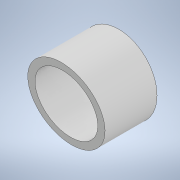
# Autodesk Inventor part: 20220612_仮筒
Saved by Autodesk Inventor 2020 (Build 240168000, 168)
## iProperties
Created: 2022-06-12
Part Number: 20220612_仮筒
Material: 一般
Document SubType Name: Modeling
Designer: Naggy
Density: 1 g/cm^3
Appearance: 既定
Author: Naggy
Autodesk Inventor part; units mm, degrees
ref_plane "YZ Plane" through (0, 0, 0) normal (1, 0, 0) x (0, 1, 0)
ref_plane "XZ Plane" through (0, 0, 0) normal (0, 1, 0) x (-1, 0, 0)
ref_plane "XY Plane" through (0, 0, 0) normal (0, 0, 1) x (1, 0, 0)
sketch "スケッチ1" plane through (0, 0, 0) normal (0, 0, 1) x (1, 0, 0)
  circle A0 centre (0, 0) radius 40
  dimension "d0" = 80
  constraints: 1 centre point, 1 coincident
  measures "d0" diameter of A0
extrude "押し出し1" add sketch "スケッチ1" along normal blind 60
sketch "スケッチ2" plane through (0, 0, 60) normal (0, 0, 1) x (1, 0, 0)
  circle A0 centre (0, 0) radius 32.5
  dimension "d3" = 65
  constraints: 1 centre point, 1 coincident
  measures "d3" diameter of A0
extrude "押し出し2" cut sketch "スケッチ2" against normal blind 60
sketch "スケッチ3" plane through (0, 0, 0) normal (1, 0, 0) x (0, 1, 0)
  line L0 (40, 0) -> (40, 60) projected
  line L1 (40, 60) -> (-40, 49.2831)
  line L2 (-40, 0) -> (-40, 60) projected
  line L3 (40, 60) -> (-40, 60) projected
  line L4 (40, 60) -> (-40, 60)
  line L5 (-40, 60) -> (-40, 49.2831)
  point P0 (0, 0)
  constraints: 6 end point, 2 collinear, 2 point on line
extrude "押し出し3" cut sketch "スケッチ3" against normal mid plane 80
sketch "スケッチ4" plane through (0, 0, 0) normal (0, 0, 1) x (1, 0, 0)
  line L0 (-32.5, -6.5) -> (32.5, -6.5)
  line L1 (32.5, -6.5) -> (32.5, 6.5)
  line L2 (32.5, 6.5) -> (-32.5, 6.5)
  line L3 (-32.5, 6.5) -> (-32.5, -6.5)
  line L4 (-32.5, -6.5) -> (32.5, 6.5) construction
  line L5 (32.5, -6.5) -> (-32.5, 6.5) construction
  point P0 (0, 0)
  dimension "d8" = 13
  dimension "d9" = 65
  constraints: 12 end point, 2 midpoint, 2 parallel, 1 horizontal, 1 perpendicular
  measures "d8" distance between parallel lines of L0 L2
  measures "d9" distance between parallel lines of L1 L3
extrude "押し出し4" add sketch "スケッチ4" along normal blind 3
sketch "スケッチ5" plane through (0, 0, 0) normal (0, 0, -1) x (-1, 0, 0)
  point P0 (0, 0)
  point P1 (-20, 0)
  point P2 (20, 0)
  dimension "d12" = 20
  dimension "d13" = 20
  measures "d12" distance of point (-20, 0) point (0, 0)
  measures "d13" distance of point (20, 0) point (0, 0)
hole "穴1" at (20, 0, 0) at (-20, 0, 0) direction (0, 0, 1) diameter 3.2 depth 15 tip angle 118
sketch "スケッチ6" plane through (0, 0, 0) normal (0, 0, -1) x (-1, 0, 0)
  point P0 (0, 0)
  point P1 (0, 0)
  constraints: 1 coincident
hole "穴2" at (0, 0, 0) direction (0, 0, 1) diameter 1.5 depth 15 tip angle 118
sketch "スケッチ7" plane through (0, 0, 0) normal (0, 0, -1) x (-1, 0, 0)
  point P0 (0, 0)
  point P1 (-8.3, 0)
  point P2 (8.3, 0)
  dimension "d28" = 8.3
  dimension "d29" = 8.3
  measures "d28" distance of point (-8.3, 0) point (0, 0)
  measures "d29" distance of point (8.3, 0) point (0, 0)
hole "穴3" at (8.3, 0, 0) at (-8.3, 0, 0) direction (0, 0, 1) diameter 3.2 depth 8.8 tip angle 118
